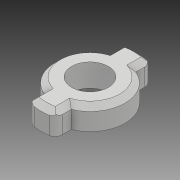
# Autodesk Inventor part: conecter
Saved by Autodesk Inventor 2018 (Build 220112000, 112)
## iProperties
Created: 2019-02-27
Part Number: conecter
Material: 一般
Document SubType Name: Modeling
Designer: ku_sk
Density: 1 g/cm^3
Appearance: 既定
Author: ku_sk
Autodesk Inventor part; units mm, degrees
ref_plane "YZ Plane" through (0, 0, 0) normal (1, 0, 0) x (0, 1, 0)
ref_plane "XZ Plane" through (0, 0, 0) normal (0, 1, 0) x (-1, 0, 0)
ref_plane "XY Plane" through (0, 0, 0) normal (0, 0, 1) x (1, 0, 0)
sketch "スケッチ1" plane through (0, 0, 0) normal (0, 0, 1) x (1, 0, 0)
  circle A0 centre (0, 0) radius 10
  dimension "d0" = 20
  constraints: 1 centre point, 1 coincident
  measures "d0" diameter of A0
extrude "押し出し1" add sketch "スケッチ1" along normal blind 6.5
sketch "スケッチ2" plane through (0, 0, 0) normal (0, 0, -1) x (-1, 0, 0)
  arc A0 (3.85, 13.4602) -> (-3.85, 13.4602) centre (0, 0) ccw
  arc A1 (-3.85, -13.4602) -> (3.85, -13.4602) centre (0, 0) ccw
  circle A2 centre (0, 0) radius 10 projected
  line L0 (-3.85, 13.4602) -> (-3.85, -13.4602)
  line L1 (3.85, -13.4602) -> (3.85, 13.4602)
  line L2 (0, -19.6) -> (0, 19.6) projected
  line L3 (14, 0) -> (-14, 0) projected
  point P0 (0, 14)
  point P1 (0, -14)
  point P2 (-3.85, 0)
  dimension "d3" = 14
  dimension "d4" = 7.7
  constraints: 6 point on circle, 4 end point, 3 point on line, 2 centre point, 2 concentric, 1 midpoint, 1 parallel
  measures "d3" radius of A0
  measures "d4" distance between parallel lines of L1 L0
extrude "押し出し2" add sketch "スケッチ2" against normal up to surface (6.5 mm away) contours L1 A2 L2 A0 | L2 A2 L0 A0 | L1 L3 L2 A2 | L2 L3 L0 A2 | L1 A2 L2 L3 | L2 A2 L0 L3 | L1 A1 L2 A2 | L2 A1 L0 A2
chamfer "面取り1" distance 1.5 angle 45 8 edges at (-10, 0, 6.5) (10, 0, 6.5) (-3.85, 11.3447, 6.5) (0, 14, 6.5) (3.85, 11.3447, 6.5) (3.85, -11.3447, 6.5) (0, -14, 6.5) (-3.85, -11.3447, 6.5)
fillet "フィレット1" radius 2 4 edges at (-3.85, -13.4602, 2.5) (3.85, -13.4602, 2.5) (3.85, 13.4602, 2.5) (-3.85, 13.4602, 2.5)
sketch "スケッチ3" plane through (0, 0, 6.5) normal (0, 0, 1) x (1, 0, 0)
  circle A0 centre (0, 0) radius 5.25
  dimension "d11" = 10.5
  constraints: 1 centre point, 1 coincident
  measures "d11" diameter of A0
extrude "押し出し3" cut sketch "スケッチ3" against normal up to surface (6.5 mm away)
